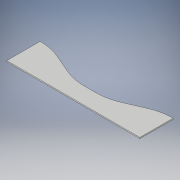
# Autodesk Inventor part: type7_base
Saved by Autodesk Inventor 2018.1 (Build 221171000, 171)
## iProperties
Created: 2017-11-03
Part Number: type7_base
Material: 一般
Document SubType Name: Modeling
Designer: ku_sk
Density: 1 g/cm^3
Appearance: 既定
Author: ku_sk
Autodesk Inventor part; units mm, degrees
ref_plane "YZ Plane" through (0, 0, 0) normal (1, 0, 0) x (0, 1, 0)
ref_plane "XZ Plane" through (0, 0, 0) normal (0, 1, 0) x (-1, 0, 0)
ref_plane "XY Plane" through (0, 0, 0) normal (0, 0, 1) x (1, 0, 0)
sketch "スケッチ1" plane through (0, 0, 0) normal (0, 1, 0) x (-1, 0, 0)
  line L0 (600, -150) -> (-600, -150)
  line L1 (-600, -150) -> (-600, 150)
  line L2 (-600, 150) -> (600, 150)
  line L3 (600, 150) -> (600, -150)
  line L4 (0, -210) -> (0, 210) projected
  line L5 (840, 0) -> (-840, 0) projected
  point P0 (0, 0)
  point P1 (0, -150)
  point P2 (600, 0)
  dimension "d0" = 1200
  dimension "d1" = 300
  constraints: 8 end point, 2 midpoint, 2 parallel, 2 point on line, 1 horizontal, 1 perpendicular
  measures "d0" distance of L0.start L0.end
  measures "d1" distance of L0.end L1.end
extrude "押し出し1" add sketch "スケッチ1" along normal blind 10
sketch "スケッチ2" plane through (0, 10, 0) normal (0, 1, 0) x (1, 0, 0)
  line L0 (0, 210) -> (0, -210) projected
  line L1 (0, 0) -> (150, 0)
  line L2 (150, 0) -> (500, 150)
  line L3 (600, 150) -> (-600, 150) projected
  line L4 (0, 0) -> (-150, 0)
  line L5 (-150, 0) -> (-500, 150)
  line L6 (600, -150) -> (600, 150) projected
  line L7 (-500, 150) -> (500, 150)
  line L8 (-600, -150) -> (600, -150) projected
  dimension "d5" = 150
  dimension "d6" = 100
  dimension "d10" = 150
  constraints: 10 end point, 2 symmetric about line, 1 collinear, 1 horizontal, 1 midpoint, 1 point on line
  measures "d5" distance of L1.start L1.end
  measures "d6" distance from line of L6 L2.end
  measures "d10" distance between parallel lines of L8 L1
extrude "押し出し2" cut sketch "スケッチ2" against normal through all contours L3 L2 L1 L0 | L0 L4 L5 L3
fillet "フィレット1" radius 500 4 edges at (-500, 5, -150) (-150, 5, 0) (150, 5, 0) (500, 5, -150)
